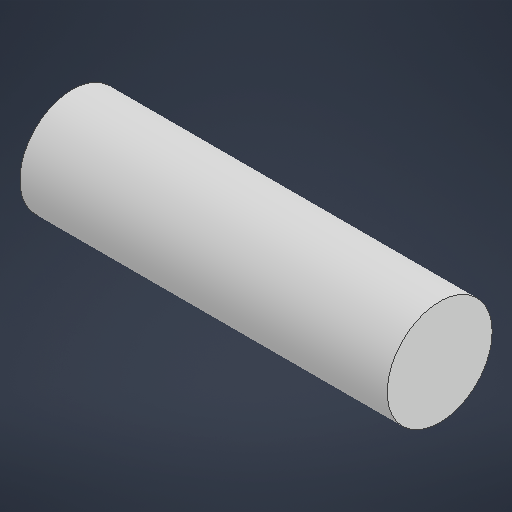
# Autodesk Inventor part: P_Spritze_60ml
Saved by Autodesk Inventor 2026 (Build 300175000, 175)
## iProperties
Created: 2025-04-25
Part Number: P_Spritze_60ml
Material: Generisch
Document SubType Name: Modeling
Designer: FAL
Density: 1 g/cm^3
Appearance: Vorgabe
Author: FAL
Autodesk Inventor part; units mm, degrees
ref_plane "YZ Plane" through (0, 0, 0) normal (1, 0, 0) x (0, 1, 0)
ref_plane "XZ Plane" through (0, 0, 0) normal (0, 1, 0) x (-1, 0, 0)
ref_plane "XY Plane" through (0, 0, 0) normal (0, 0, 1) x (1, 0, 0)
sketch "Skizze2" plane through (0, 0, 0) normal (0, 0, 1) x (1, 0, 0)
  line L0 (0, 0) -> (50, 0) construction
  line L1 (0, 0) -> (0, 7.1423)
  line L2 (0, 7.1423) -> (50, 7.1423)
  line L3 (50, 7.1423) -> (50, 0)
  line L4 (0.6905, 6.4517) -> (0.6905, 0)
  line L5 (49.3095, 0) -> (49.3095, 6.4517)
  line L6 (49.3095, 6.4517) -> (0.6905, 6.4517)
  line L7 (0, 0) -> (0.6905, 0)
  line L8 (49.3095, 0) -> (50, 0)
  dimension "d0" = 50
  constraints: 18 end point, 6 perpendicular, 3 horizontal, 2 point on line, 1 vertical, 1 other
  measures "d0" distance of L0.start L0.end
revolve "Umdrehung1" add sketch "Skizze2" angle 360 about axis through (0, 0, 0) along (1, 0, 0)
